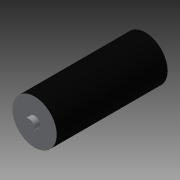
# Autodesk Inventor part: Shooter_RollerTop
Saved by Autodesk Inventor 2014 (Build 180170000, 170)
## iProperties
Created: 2016-01-26
Part Number: Shooter_RollerTop
Material: Generic
Document SubType Name: Modeling
Designer: shawnsargent
Density: 1 g/cm^3
Appearance: Default
Author: shawnsargent
Autodesk Inventor part; units mm, degrees
ref_plane "YZ Plane" through (0, 0, 0) normal (1, 0, 0) x (0, 1, 0)
ref_plane "XZ Plane" through (0, 0, 0) normal (0, 1, 0) x (-1, 0, 0)
ref_plane "XY Plane" through (0, 0, 0) normal (0, 0, 1) x (1, 0, 0)
sketch "Sketch1" plane through (0, 0, 0) normal (0, 0, 1) x (1, 0, 0)
  circle A0 centre (0, 0) radius 31.75
  dimension "d0" = 63.5
  constraints: 1 centre point, 1 coincident
  measures "d0" diameter of A0
extrude "Extrusion1" add sketch "Sketch1" along normal blind 82.55
sketch "Sketch2" plane through (0, 0, 82.55) normal (0, 0, 1) x (1, 0, 0)
  circle A0 centre (0, 0) radius 31.75 projected
  circle A1 centre (0, 0) radius 14.859
  dimension "d3" = 29.718
  constraints: 1 centre point, 1 coincident
  measures "d3" diameter of A1
extrude "Extrusion2" add sketch "Sketch2" along normal blind 6.35 contours A1
sketch "Sketch3" plane through (0, 0, 0) normal (0, 0, -1) x (-1, 0, 0)
  circle A0 centre (0, 0) radius 31.75 projected
  circle A1 centre (0, 0) radius 12.7
  dimension "d6" = 25.4
  constraints: 1 centre point, 1 coincident
  measures "d6" diameter of A1
extrude "Extrusion3" add sketch "Sketch3" along normal blind 12.7 contours A1
sketch "Sketch4" plane through (0, 0, -12.7) normal (0, 0, -1) x (-1, 0, 0)
  circle A0 centre (0, 0) radius 12.7 projected
  circle A1 centre (0, 0) radius 50.8
  dimension "d9" = 101.6
  constraints: 1 centre point, 1 coincident
  measures "d9" diameter of A1
extrude "Extrusion4" add sketch "Sketch4" along normal blind 254 contours A0 | A1
sketch "Sketch5" plane through (0, 0, -266.7) normal (0, 0, -1) x (-1, 0, 0)
  circle A0 centre (0, 0) radius 50.8 projected
  circle A1 centre (0, 0) radius 12.7
  dimension "d12" = 25.4
  constraints: 1 centre point, 1 coincident
  measures "d12" diameter of A1
extrude "Extrusion5" add sketch "Sketch5" along normal blind 12.7 contours A1
sketch "Sketch7" plane through (0, 0, 88.9) normal (0, 0, 1) x (1, 0, 0)
  circle A0 centre (0, 0) radius 14.859 projected
  circle A1 centre (0, 0) radius 117.3057
  constraints: 1 centre point, 1 coincident
extrude "Extrusion6" cut sketch "Sketch7" against normal blind 88.9 contours A0 | A1
body "Solid1"
